Autodesk Inventor part; units mm, degrees
(part 2 of 3)
  line L844 (-43.6734, 26.1204) -> (-43.9834, 26.1204) projected
  line L845 (-43.9834, 26.1204) -> (-43.9834, 25.7204) projected
  line L846 (-43.9834, 25.7204) -> (-43.6734, 25.7204) projected
  line L847 (-43.6734, 25.7204) -> (-43.6734, 25.3204) projected
  line L848 (-43.6734, 25.3204) -> (-43.9834, 25.3204) projected
  line L849 (-43.9834, 25.3204) -> (-43.9834, 24.9204) projected
  line L850 (-43.9834, 24.9204) -> (-43.6734, 24.9204) projected
  line L851 (-43.6734, 24.9204) -> (-43.6734, 24.5204) projected
  line L852 (-43.6734, 24.5204) -> (-43.9834, 24.5204) projected
  line L853 (-43.9834, 24.5204) -> (-43.9834, 24.1204) projected
  line L854 (-43.9834, 24.1204) -> (-43.6734, 24.1204) projected
  line L855 (-43.6734, 24.1204) -> (-43.6734, 23.7204) projected
  line L856 (-43.6734, 23.7204) -> (-43.9834, 23.7204) projected
  line L857 (-43.9834, 23.7204) -> (-43.9834, 23.4704) projected
  arc A41 (-44.5384, 22.5149) -> (-43.9834, 23.4704) centre (-45.0834, 23.4704) ccw projected
  line L858 (-44.5384, 22.5149) -> (-44.5384, 22.4454) projected
  line L859 (-44.5384, 22.4454) -> (-44.6842, 22.4454) projected
  line L860 (-25.2834, -31.9046) -> (-25.2834, -32.3046) projected
  line L861 (-25.2834, -32.3046) -> (-24.6634, -32.3046) projected
  line L862 (-24.6634, -32.3046) -> (-24.6634, -32.7046) projected
  line L863 (-24.6634, -32.7046) -> (-25.286, -32.7046) projected
  arc A42 (-25.5349, -33.3296) -> (-25.286, -32.7046) centre (-26.3834, -32.6296) ccw projected
  line L864 (-25.5349, -33.3296) -> (-25.5284, -33.3296) projected
  line L865 (-25.5284, -33.3296) -> (-25.5284, -33.9796) projected
  line L866 (-25.5284, -33.9796) -> (-27.1284, -33.9796) projected
  line L867 (-27.1284, -33.9796) -> (-27.1284, -33.4389) projected
  arc A43 (-27.4808, -32.7046) -> (-27.1284, -33.4389) centre (-26.3834, -32.6296) ccw projected
  line L868 (-27.4808, -32.7046) -> (-27.9934, -32.7046) projected
  line L869 (-27.9934, -32.7046) -> (-27.9934, -32.3046) projected
  line L870 (-27.9934, -32.3046) -> (-27.4834, -32.3046) projected
  line L871 (-27.4834, -32.3046) -> (-27.4834, -31.9046) projected
  line L872 (-27.4834, -31.9046) -> (-27.9934, -31.9046) projected
  line L873 (-27.9934, -31.9046) -> (-27.9934, -31.5046) projected
  line L874 (-27.9934, -31.5046) -> (-27.4834, -31.5046) projected
  line L875 (-27.4834, -31.5046) -> (-27.4834, -31.1046) projected
  line L876 (-27.4834, -31.1046) -> (-27.9934, -31.1046) projected
  line L877 (-27.9934, -31.1046) -> (-27.9934, -30.7046) projected
  line L878 (-27.9934, -30.7046) -> (-27.4834, -30.7046) projected
  line L879 (-27.4834, -30.7046) -> (-27.4834, -30.3046) projected
  line L880 (-27.4834, -30.3046) -> (-27.9934, -30.3046) projected
  line L881 (-27.9934, -30.3046) -> (-27.9934, -29.9046) projected
  line L882 (-27.9934, -29.9046) -> (-27.4834, -29.9046) projected
  line L883 (-27.4834, -29.9046) -> (-27.4834, -29.5046) projected
  line L884 (-27.4834, -29.5046) -> (-27.9934, -29.5046) projected
  line L885 (-27.9934, -29.5046) -> (-27.9934, -29.1046) projected
  line L886 (-27.9934, -29.1046) -> (-27.4834, -29.1046) projected
  line L887 (-27.4834, -29.1046) -> (-27.4834, -28.7046) projected
  line L888 (-27.4834, -28.7046) -> (-27.9934, -28.7046) projected
  line L889 (-27.9934, -28.7046) -> (-27.9934, -28.3046) projected
  line L890 (-27.9934, -28.3046) -> (-27.4834, -28.3046) projected
  line L891 (-27.4834, -28.3046) -> (-27.4834, -27.9046) projected
  line L892 (-27.4834, -27.9046) -> (-27.9934, -27.9046) projected
  line L893 (-27.9934, -27.9046) -> (-27.9934, -27.5046) projected
  line L894 (-27.9934, -27.5046) -> (-27.4834, -27.5046) projected
  line L895 (-27.4834, -27.5046) -> (-27.4834, -27.1046) projected
  line L896 (-27.4834, -27.1046) -> (-27.9934, -27.1046) projected
  line L897 (-27.9934, -27.1046) -> (-27.9934, -26.7046) projected
  line L898 (-27.9934, -26.7046) -> (-27.4831, -26.7046) projected
  arc A44 (-27.1284, -25.9203) -> (-27.4831, -26.7046) centre (-26.3834, -26.7296) ccw projected
  line L899 (-27.1284, -25.9203) -> (-27.1284, -25.4296) projected
  line L900 (-27.1284, -25.4296) -> (-25.5284, -25.4296) projected
  line L901 (-25.5284, -25.4296) -> (-25.5284, -26.0375) projected
  arc A45 (-25.2837, -26.7046) -> (-25.5284, -26.0375) centre (-26.3834, -26.7296) ccw projected
  line L902 (-25.2837, -26.7046) -> (-24.6634, -26.7046) projected
  line L903 (-24.6634, -26.7046) -> (-24.6634, -27.1046) projected
  line L904 (-24.6634, -27.1046) -> (-25.2834, -27.1046) projected
  line L905 (-25.2834, -27.1046) -> (-25.2834, -27.5046) projected
  line L906 (-25.2834, -27.5046) -> (-24.6634, -27.5046) projected
  line L907 (-24.6634, -27.5046) -> (-24.6634, -27.9046) projected
  line L908 (-24.6634, -27.9046) -> (-25.2834, -27.9046) projected
  line L909 (-25.2834, -27.9046) -> (-25.2834, -28.3046) projected
  line L910 (-25.2834, -28.3046) -> (-24.6634, -28.3046) projected
  line L911 (-24.6634, -28.3046) -> (-24.6634, -28.7046) projected
  line L912 (-24.6634, -28.7046) -> (-25.2834, -28.7046) projected
  line L913 (-25.2834, -28.7046) -> (-25.2834, -29.1046) projected
  line L914 (-25.2834, -29.1046) -> (-24.6634, -29.1046) projected
  line L915 (-24.6634, -29.1046) -> (-24.6634, -29.5046) projected
  line L916 (-24.6634, -29.5046) -> (-25.2834, -29.5046) projected
  line L917 (-25.2834, -29.5046) -> (-25.2834, -29.9046) projected
  line L918 (-25.2834, -29.9046) -> (-24.6634, -29.9046) projected
  line L919 (-24.6634, -29.9046) -> (-24.6634, -30.3046) projected
  line L920 (-24.6634, -30.3046) -> (-25.2834, -30.3046) projected
  line L921 (-25.2834, -30.3046) -> (-25.2834, -30.7046) projected
  line L922 (-25.2834, -30.7046) -> (-24.6634, -30.7046) projected
  line L923 (-24.6634, -30.7046) -> (-24.6634, -31.1046) projected
  line L924 (-24.6634, -31.1046) -> (-25.2834, -31.1046) projected
  line L925 (-25.2834, -31.1046) -> (-25.2834, -31.5046) projected
  line L926 (-25.2834, -31.5046) -> (-24.6634, -31.5046) projected
  line L927 (-24.6634, -31.5046) -> (-24.6634, -31.9046) projected
  line L928 (-24.6634, -31.9046) -> (-25.2834, -31.9046) projected
  arc A46 (-26.6166, 3.6954) -> (-26.1502, 3.6954) centre (-26.3834, 4.7704) ccw projected
  line L929 (-26.6166, 3.6954) -> (-27.2859, 3.6954) projected
  line L930 (-27.2859, 3.6954) -> (-27.2859, 4.1415) projected
  arc A47 (-27.4834, 4.7704) -> (-27.2859, 4.1415) centre (-26.3834, 4.7704) ccw projected
  line L931 (-27.4834, 4.7704) -> (-27.4834, 4.9704) projected
  line L932 (-27.4834, 4.9704) -> (-28.1509, 4.9704) projected
  line L933 (-28.1509, 4.9704) -> (-28.1509, 5.3704) projected
  line L934 (-28.1509, 5.3704) -> (-27.4834, 5.3704) projected
  line L935 (-27.4834, 5.3704) -> (-27.4834, 5.7704) projected
  line L936 (-27.4834, 5.7704) -> (-28.1509, 5.7704) projected
  line L937 (-28.1509, 5.7704) -> (-28.1509, 6.1704) projected
  line L938 (-28.1509, 6.1704) -> (-27.4834, 6.1704) projected
  line L939 (-27.4834, 6.1704) -> (-27.4834, 6.5704) projected
  line L940 (-27.4834, 6.5704) -> (-28.1509, 6.5704) projected
  line L941 (-28.1509, 6.5704) -> (-28.1509, 6.9704) projected
  line L942 (-28.1509, 6.9704) -> (-27.4834, 6.9704) projected
  line L943 (-27.4834, 6.9704) -> (-27.4834, 7.3704) projected
  line L944 (-27.4834, 7.3704) -> (-28.1509, 7.3704) projected
  line L945 (-28.1509, 7.3704) -> (-28.1509, 7.7704) projected
  line L946 (-28.1509, 7.7704) -> (-27.4834, 7.7704) projected
  line L947 (-27.4834, 7.7704) -> (-27.4834, 8.1704) projected
  line L948 (-27.4834, 8.1704) -> (-28.1509, 8.1704) projected
  line L949 (-28.1509, 8.1704) -> (-28.1509, 8.5704) projected
  line L950 (-28.1509, 8.5704) -> (-27.4834, 8.5704) projected
  line L951 (-27.4834, 8.5704) -> (-27.4834, 8.9704) projected
  line L952 (-27.4834, 8.9704) -> (-28.1509, 8.9704) projected
  line L953 (-28.1509, 8.9704) -> (-28.1509, 9.3704) projected
  line L954 (-28.1509, 9.3704) -> (-27.4834, 9.3704) projected
  line L955 (-27.4834, 9.3704) -> (-27.4834, 9.7704) projected
  line L956 (-27.4834, 9.7704) -> (-28.1509, 9.7704) projected
  line L957 (-28.1509, 9.7704) -> (-28.1509, 10.1704) projected
  line L958 (-28.1509, 10.1704) -> (-27.4834, 10.1704) projected
  line L959 (-27.4834, 10.1704) -> (-27.4834, 10.5704) projected
  line L960 (-27.4834, 10.5704) -> (-28.1509, 10.5704) projected
  line L961 (-28.1509, 10.5704) -> (-28.1509, 10.9704) projected
  line L962 (-28.1509, 10.9704) -> (-27.4417, 10.9704) projected
  arc A48 (-26.9787, 11.5954) -> (-27.4417, 10.9704) centre (-26.3834, 10.6704) ccw projected
  line L963 (-26.9787, 11.5954) -> (-27.2859, 11.5954) projected
  line L964 (-27.2859, 11.5954) -> (-27.2859, 12.2454) projected
  line L965 (-27.2859, 12.2454) -> (-25.6859, 12.2454) projected
  line L966 (-25.6859, 12.2454) -> (-25.6859, 11.5954) projected
  line L967 (-25.6859, 11.5954) -> (-25.7881, 11.5954) projected
  arc A49 (-25.3251, 10.9704) -> (-25.7881, 11.5954) centre (-26.3834, 10.6704) ccw projected
  line L968 (-25.3251, 10.9704) -> (-24.8209, 10.9704) projected
  line L969 (-24.8209, 10.9704) -> (-24.8209, 10.5704) projected
  line L970 (-24.8209, 10.5704) -> (-25.2834, 10.5704) projected
  line L971 (-25.2834, 10.5704) -> (-25.2834, 10.1704) projected
  line L972 (-25.2834, 10.1704) -> (-24.8209, 10.1704) projected
  line L973 (-24.8209, 10.1704) -> (-24.8209, 9.7704) projected
  line L974 (-24.8209, 9.7704) -> (-25.2834, 9.7704) projected
  line L975 (-25.2834, 9.7704) -> (-25.2834, 9.3704) projected
  line L976 (-25.2834, 9.3704) -> (-24.8209, 9.3704) projected
  line L977 (-24.8209, 9.3704) -> (-24.8209, 8.9704) projected
  line L978 (-24.8209, 8.9704) -> (-25.2834, 8.9704) projected
  line L979 (-25.2834, 8.9704) -> (-25.2834, 8.5704) projected
  line L980 (-25.2834, 8.5704) -> (-24.8209, 8.5704) projected
  line L981 (-24.8209, 8.5704) -> (-24.8209, 8.1704) projected
  line L982 (-24.8209, 8.1704) -> (-25.2834, 8.1704) projected
  line L983 (-25.2834, 8.1704) -> (-25.2834, 7.7704) projected
  line L984 (-25.2834, 7.7704) -> (-24.8209, 7.7704) projected
  line L985 (-24.8209, 7.7704) -> (-24.8209, 7.3704) projected
  line L986 (-24.8209, 7.3704) -> (-25.2834, 7.3704) projected
  line L987 (-25.2834, 7.3704) -> (-25.2834, 6.9704) projected
  line L988 (-25.2834, 6.9704) -> (-24.8209, 6.9704) projected
  line L989 (-24.8209, 6.9704) -> (-24.8209, 6.5704) projected
  line L990 (-24.8209, 6.5704) -> (-25.2834, 6.5704) projected
  line L991 (-25.2834, 6.5704) -> (-25.2834, 6.1704) projected
  line L992 (-25.2834, 6.1704) -> (-24.8209, 6.1704) projected
  line L993 (-24.8209, 6.1704) -> (-24.8209, 5.7704) projected
  line L994 (-24.8209, 5.7704) -> (-25.2834, 5.7704) projected
  line L995 (-25.2834, 5.7704) -> (-25.2834, 5.3704) projected
  line L996 (-25.2834, 5.3704) -> (-24.8209, 5.3704) projected
  line L997 (-24.8209, 5.3704) -> (-24.8209, 4.9704) projected
  line L998 (-24.8209, 4.9704) -> (-25.2834, 4.9704) projected
  line L999 (-25.2834, 4.9704) -> (-25.2834, 4.7704) projected
  arc A50 (-25.6859, 3.9198) -> (-25.2834, 4.7704) centre (-26.3834, 4.7704) ccw projected
  line L1000 (-25.6859, 3.9198) -> (-25.6859, 3.6954) projected
  line L1001 (-25.6859, 3.6954) -> (-26.1502, 3.6954) projected
  arc A51 (-26.7113, 22.4204) -> (-26.0555, 22.4204) centre (-26.3834, 23.4704) ccw projected
  line L1002 (-26.7113, 22.4204) -> (-27.0884, 22.4204) projected
  line L1003 (-27.0884, 22.4204) -> (-27.0884, 22.626) projected
  arc A52 (-27.4834, 23.4704) -> (-27.0884, 22.626) centre (-26.3834, 23.4704) ccw projected
  line L1004 (-27.4834, 23.4704) -> (-27.4834, 23.6954) projected
  line L1005 (-27.4834, 23.6954) -> (-27.9534, 23.6954) projected
  line L1006 (-27.9534, 23.6954) -> (-27.9534, 24.0954) projected
  line L1007 (-27.9534, 24.0954) -> (-27.4834, 24.0954) projected
  line L1008 (-27.4834, 24.0954) -> (-27.4834, 24.4954) projected
  line L1009 (-27.4834, 24.4954) -> (-27.9534, 24.4954) projected
  line L1010 (-27.9534, 24.4954) -> (-27.9534, 24.8954) projected
  line L1011 (-27.9534, 24.8954) -> (-27.4834, 24.8954) projected
  line L1012 (-27.4834, 24.8954) -> (-27.4834, 25.2954) projected
  line L1013 (-27.4834, 25.2954) -> (-27.9534, 25.2954) projected
  line L1014 (-27.9534, 25.2954) -> (-27.9534, 25.6954) projected
  line L1015 (-27.9534, 25.6954) -> (-27.4834, 25.6954) projected
  line L1016 (-27.4834, 25.6954) -> (-27.4834, 26.0954) projected
  line L1017 (-27.4834, 26.0954) -> (-27.9534, 26.0954) projected
  line L1018 (-27.9534, 26.0954) -> (-27.9534, 26.4954) projected
  line L1019 (-27.9534, 26.4954) -> (-27.4834, 26.4954) projected
  line L1020 (-27.4834, 26.4954) -> (-27.4834, 26.8954) projected
  line L1021 (-27.4834, 26.8954) -> (-27.9534, 26.8954) projected
  line L1022 (-27.9534, 26.8954) -> (-27.9534, 27.2954) projected
  line L1023 (-27.9534, 27.2954) -> (-27.4834, 27.2954) projected
  line L1024 (-27.4834, 27.2954) -> (-27.4834, 27.6954) projected
  line L1025 (-27.4834, 27.6954) -> (-27.9534, 27.6954) projected
  line L1026 (-27.9534, 27.6954) -> (-27.9534, 28.0954) projected
  line L1027 (-27.9534, 28.0954) -> (-27.4834, 28.0954) projected
  line L1028 (-27.4834, 28.0954) -> (-27.4834, 28.4954) projected
  line L1029 (-27.4834, 28.4954) -> (-27.9534, 28.4954) projected
  line L1030 (-27.9534, 28.4954) -> (-27.9534, 28.8954) projected
  line L1031 (-27.9534, 28.8954) -> (-27.4834, 28.8954) projected
  line L1032 (-27.4834, 28.8954) -> (-27.4834, 29.2954) projected
  line L1033 (-27.4834, 29.2954) -> (-27.9534, 29.2954) projected
  line L1034 (-27.9534, 29.2954) -> (-27.9534, 29.6954) projected
  line L1035 (-27.9534, 29.6954) -> (-27.4343, 29.6954) projected
  arc A53 (-26.9379, 30.3204) -> (-27.4343, 29.6954) centre (-26.3834, 29.3704) ccw projected
  line L1036 (-26.9379, 30.3204) -> (-27.0884, 30.3204) projected
  line L1037 (-27.0884, 30.3204) -> (-27.0884, 30.9704) projected
  line L1038 (-27.0884, 30.9704) -> (-25.4884, 30.9704) projected
  line L1039 (-25.4884, 30.9704) -> (-25.4884, 30.3204) projected
  line L1040 (-25.4884, 30.3204) -> (-25.8289, 30.3204) projected
  arc A54 (-25.3325, 29.6954) -> (-25.8289, 30.3204) centre (-26.3834, 29.3704) ccw projected
  line L1041 (-25.3325, 29.6954) -> (-24.6234, 29.6954) projected
  line L1042 (-24.6234, 29.6954) -> (-24.6234, 29.2954) projected
  line L1043 (-24.6234, 29.2954) -> (-25.2834, 29.2954) projected
  line L1044 (-25.2834, 29.2954) -> (-25.2834, 28.8954) projected
  line L1045 (-25.2834, 28.8954) -> (-24.6234, 28.8954) projected
  line L1046 (-24.6234, 28.8954) -> (-24.6234, 28.4954) projected
  line L1047 (-24.6234, 28.4954) -> (-25.2834, 28.4954) projected
  line L1048 (-25.2834, 28.4954) -> (-25.2834, 28.0954) projected
  line L1049 (-25.2834, 28.0954) -> (-24.6234, 28.0954) projected
  line L1050 (-24.6234, 28.0954) -> (-24.6234, 27.6954) projected
  line L1051 (-24.6234, 27.6954) -> (-25.2834, 27.6954) projected
  line L1052 (-25.2834, 27.6954) -> (-25.2834, 27.2954) projected
  line L1053 (-25.2834, 27.2954) -> (-24.6234, 27.2954) projected
  line L1054 (-24.6234, 27.2954) -> (-24.6234, 26.8954) projected
  line L1055 (-24.6234, 26.8954) -> (-25.2834, 26.8954) projected
  line L1056 (-25.2834, 26.8954) -> (-25.2834, 26.4954) projected
  line L1057 (-25.2834, 26.4954) -> (-24.6234, 26.4954) projected
  line L1058 (-24.6234, 26.4954) -> (-24.6234, 26.0954) projected
  line L1059 (-24.6234, 26.0954) -> (-25.2834, 26.0954) projected
  line L1060 (-25.2834, 26.0954) -> (-25.2834, 25.6954) projected
  line L1061 (-25.2834, 25.6954) -> (-24.6234, 25.6954) projected
  line L1062 (-24.6234, 25.6954) -> (-24.6234, 25.2954) projected
  line L1063 (-24.6234, 25.2954) -> (-25.2834, 25.2954) projected
  line L1064 (-25.2834, 25.2954) -> (-25.2834, 24.8954) projected
  line L1065 (-25.2834, 24.8954) -> (-24.6234, 24.8954) projected
  line L1066 (-24.6234, 24.8954) -> (-24.6234, 24.4954) projected
  line L1067 (-24.6234, 24.4954) -> (-25.2834, 24.4954) projected
  line L1068 (-25.2834, 24.4954) -> (-25.2834, 24.0954) projected
  line L1069 (-25.2834, 24.0954) -> (-24.6234, 24.0954) projected
  line L1070 (-24.6234, 24.0954) -> (-24.6234, 23.6954) projected
  line L1071 (-24.6234, 23.6954) -> (-25.2834, 23.6954) projected
  line L1072 (-25.2834, 23.6954) -> (-25.2834, 23.4704) projected
  arc A55 (-25.4884, 22.8309) -> (-25.2834, 23.4704) centre (-26.3834, 23.4704) ccw projected
  line L1073 (-25.4884, 22.8309) -> (-25.4884, 22.4204) projected
  line L1074 (-25.4884, 22.4204) -> (-26.0555, 22.4204) projected
  line L1075 (-6.5834, -31.8296) -> (-6.5834, -32.2296) projected
  line L1076 (-6.5834, -32.2296) -> (-5.8559, -32.2296) projected
  line L1077 (-5.8559, -32.2296) -> (-5.8559, -32.6296) projected
  line L1078 (-5.8559, -32.6296) -> (-6.5834, -32.6296) projected
  arc A56 (-6.7782, -33.2546) -> (-6.5834, -32.6296) centre (-7.6834, -32.6296) ccw projected
  line L1079 (-6.7782, -33.2546) -> (-6.7209, -33.2546) projected
  line L1080 (-6.7209, -33.2546) -> (-6.7209, -33.9046) projected
  line L1081 (-6.7209, -33.9046) -> (-8.3209, -33.9046) projected
  line L1082 (-8.3209, -33.9046) -> (-8.3209, -33.526) projected
  arc A57 (-8.7834, -32.6296) -> (-8.3209, -33.526) centre (-7.6834, -32.6296) ccw projected
  line L1083 (-8.7834, -32.6296) -> (-9.1859, -32.6296) projected
  line L1084 (-9.1859, -32.6296) -> (-9.1859, -32.2296) projected
  line L1085 (-9.1859, -32.2296) -> (-8.7834, -32.2296) projected
  line L1086 (-8.7834, -32.2296) -> (-8.7834, -31.8296) projected
  line L1087 (-8.7834, -31.8296) -> (-9.1859, -31.8296) projected
  line L1088 (-9.1859, -31.8296) -> (-9.1859, -31.4296) projected
  line L1089 (-9.1859, -31.4296) -> (-8.7834, -31.4296) projected
  line L1090 (-8.7834, -31.4296) -> (-8.7834, -31.0296) projected
  line L1091 (-8.7834, -31.0296) -> (-9.1859, -31.0296) projected
  line L1092 (-9.1859, -31.0296) -> (-9.1859, -30.6296) projected
  line L1093 (-9.1859, -30.6296) -> (-8.7834, -30.6296) projected
  line L1094 (-8.7834, -30.6296) -> (-8.7834, -30.2296) projected
  line L1095 (-8.7834, -30.2296) -> (-9.1859, -30.2296) projected
  line L1096 (-9.1859, -30.2296) -> (-9.1859, -29.8296) projected
  line L1097 (-9.1859, -29.8296) -> (-8.7834, -29.8296) projected
  line L1098 (-8.7834, -29.8296) -> (-8.7834, -29.4296) projected
  line L1099 (-8.7834, -29.4296) -> (-9.1859, -29.4296) projected
  line L1100 (-9.1859, -29.4296) -> (-9.1859, -29.0296) projected
  line L1101 (-9.1859, -29.0296) -> (-8.7834, -29.0296) projected
  line L1102 (-8.7834, -29.0296) -> (-8.7834, -28.6296) projected
  line L1103 (-8.7834, -28.6296) -> (-9.1859, -28.6296) projected
  line L1104 (-9.1859, -28.6296) -> (-9.1859, -28.2296) projected
  line L1105 (-9.1859, -28.2296) -> (-8.7834, -28.2296) projected
  line L1106 (-8.7834, -28.2296) -> (-8.7834, -27.8296) projected
  line L1107 (-8.7834, -27.8296) -> (-9.1859, -27.8296) projected
  line L1108 (-9.1859, -27.8296) -> (-9.1859, -27.4296) projected
  line L1109 (-9.1859, -27.4296) -> (-8.7834, -27.4296) projected
  line L1110 (-8.7834, -27.4296) -> (-8.7834, -27.0296) projected
  line L1111 (-8.7834, -27.0296) -> (-9.1859, -27.0296) projected
  line L1112 (-9.1859, -27.0296) -> (-9.1859, -26.6296) projected
  line L1113 (-9.1859, -26.6296) -> (-8.7788, -26.6296) projected
  arc A58 (-8.3209, -25.8332) -> (-8.7788, -26.6296) centre (-7.6834, -26.7296) ccw projected
  line L1114 (-8.3209, -25.8332) -> (-8.3209, -25.3546) projected
  line L1115 (-8.3209, -25.3546) -> (-6.7209, -25.3546) projected
  line L1116 (-6.7209, -25.3546) -> (-6.7209, -26.0046) projected
  line L1117 (-6.7209, -26.0046) -> (-6.8561, -26.0046) projected
  arc A59 (-6.588, -26.6296) -> (-6.8561, -26.0046) centre (-7.6834, -26.7296) ccw projected
  line L1118 (-6.588, -26.6296) -> (-5.8559, -26.6296) projected
  line L1119 (-5.8559, -26.6296) -> (-5.8559, -27.0296) projected
  line L1120 (-5.8559, -27.0296) -> (-6.5834, -27.0296) projected
  line L1121 (-6.5834, -27.0296) -> (-6.5834, -27.4296) projected
  line L1122 (-6.5834, -27.4296) -> (-5.8559, -27.4296) projected
  line L1123 (-5.8559, -27.4296) -> (-5.8559, -27.8296) projected
  line L1124 (-5.8559, -27.8296) -> (-6.5834, -27.8296) projected
  line L1125 (-6.5834, -27.8296) -> (-6.5834, -28.2296) projected
  line L1126 (-6.5834, -28.2296) -> (-5.8559, -28.2296) projected
  line L1127 (-5.8559, -28.2296) -> (-5.8559, -28.6296) projected
  line L1128 (-5.8559, -28.6296) -> (-6.5834, -28.6296) projected
  line L1129 (-6.5834, -28.6296) -> (-6.5834, -29.0296) projected
  line L1130 (-6.5834, -29.0296) -> (-5.8559, -29.0296) projected
  line L1131 (-5.8559, -29.0296) -> (-5.8559, -29.4296) projected
  line L1132 (-5.8559, -29.4296) -> (-6.5834, -29.4296) projected
  line L1133 (-6.5834, -29.4296) -> (-6.5834, -29.8296) projected
  line L1134 (-6.5834, -29.8296) -> (-5.8559, -29.8296) projected
  line L1135 (-5.8559, -29.8296) -> (-5.8559, -30.2296) projected
  line L1136 (-5.8559, -30.2296) -> (-6.5834, -30.2296) projected
  line L1137 (-6.5834, -30.2296) -> (-6.5834, -30.6296) projected
  line L1138 (-6.5834, -30.6296) -> (-5.8559, -30.6296) projected
  line L1139 (-5.8559, -30.6296) -> (-5.8559, -31.0296) projected
  line L1140 (-5.8559, -31.0296) -> (-6.5834, -31.0296) projected
  line L1141 (-6.5834, -31.0296) -> (-6.5834, -31.4296) projected
  line L1142 (-6.5834, -31.4296) -> (-5.8559, -31.4296) projected
  line L1143 (-5.8559, -31.4296) -> (-5.8559, -31.8296) projected
  line L1144 (-5.8559, -31.8296) -> (-6.5834, -31.8296) projected
  arc A60 (-8.1417, 3.7704) -> (-7.2251, 3.7704) centre (-7.6834, 4.7704) ccw projected
  line L1145 (-8.1417, 3.7704) -> (-8.4784, 3.7704) projected
  line L1146 (-8.4784, 3.7704) -> (-8.4784, 4.0102) projected
  arc A61 (-8.7834, 4.7704) -> (-8.4784, 4.0102) centre (-7.6834, 4.7704) ccw projected
  line L1147 (-8.7834, 4.7704) -> (-8.7834, 5.0454) projected
  line L1148 (-8.7834, 5.0454) -> (-9.3434, 5.0454) projected
  line L1149 (-9.3434, 5.0454) -> (-9.3434, 5.4454) projected
  line L1150 (-9.3434, 5.4454) -> (-8.7834, 5.4454) projected
  line L1151 (-8.7834, 5.4454) -> (-8.7834, 5.8454) projected
  line L1152 (-8.7834, 5.8454) -> (-9.3434, 5.8454) projected
  line L1153 (-9.3434, 5.8454) -> (-9.3434, 6.2454) projected
  line L1154 (-9.3434, 6.2454) -> (-8.7834, 6.2454) projected
  line L1155 (-8.7834, 6.2454) -> (-8.7834, 6.6454) projected
  line L1156 (-8.7834, 6.6454) -> (-9.3434, 6.6454) projected
  line L1157 (-9.3434, 6.6454) -> (-9.3434, 7.0454) projected
  line L1158 (-9.3434, 7.0454) -> (-8.7834, 7.0454) projected
  line L1159 (-8.7834, 7.0454) -> (-8.7834, 7.4454) projected
  line L1160 (-8.7834, 7.4454) -> (-9.3434, 7.4454) projected
  line L1161 (-9.3434, 7.4454) -> (-9.3434, 7.8454) projected
  line L1162 (-9.3434, 7.8454) -> (-8.7834, 7.8454) projected
  line L1163 (-8.7834, 7.8454) -> (-8.7834, 8.2454) projected
  line L1164 (-8.7834, 8.2454) -> (-9.3434, 8.2454) projected
  line L1165 (-9.3434, 8.2454) -> (-9.3434, 8.6454) projected
  line L1166 (-9.3434, 8.6454) -> (-8.7834, 8.6454) projected
  line L1167 (-8.7834, 8.6454) -> (-8.7834, 9.0454) projected
  line L1168 (-8.7834, 9.0454) -> (-9.3434, 9.0454) projected
  line L1169 (-9.3434, 9.0454) -> (-9.3434, 9.4454) projected
  line L1170 (-9.3434, 9.4454) -> (-8.7834, 9.4454) projected
  line L1171 (-8.7834, 9.4454) -> (-8.7834, 9.8454) projected
  line L1172 (-8.7834, 9.8454) -> (-9.3434, 9.8454) projected
  line L1173 (-9.3434, 9.8454) -> (-9.3434, 10.2454) projected
  line L1174 (-9.3434, 10.2454) -> (-8.7834, 10.2454) projected
  line L1175 (-8.7834, 10.2454) -> (-8.7834, 10.6454) projected
  line L1176 (-8.7834, 10.6454) -> (-9.3434, 10.6454) projected
  line L1177 (-9.3434, 10.6454) -> (-9.3434, 11.0454) projected
  line L1178 (-9.3434, 11.0454) -> (-8.7175, 11.0454) projected
  arc A62 (-8.1417, 11.6704) -> (-8.7175, 11.0454) centre (-7.6834, 10.6704) ccw projected
  line L1179 (-8.1417, 11.6704) -> (-8.4784, 11.6704) projected
  line L1180 (-8.4784, 11.6704) -> (-8.4784, 12.3204) projected
  line L1181 (-8.4784, 12.3204) -> (-6.8784, 12.3204) projected
  line L1182 (-6.8784, 12.3204) -> (-6.8784, 11.6704) projected
  line L1183 (-6.8784, 11.6704) -> (-7.2251, 11.6704) projected
  arc A63 (-6.6493, 11.0454) -> (-7.2251, 11.6704) centre (-7.6834, 10.6704) ccw projected
  line L1184 (-6.6493, 11.0454) -> (-6.0134, 11.0454) projected
  line L1185 (-6.0134, 11.0454) -> (-6.0134, 10.6454) projected
  line L1186 (-6.0134, 10.6454) -> (-6.5834, 10.6454) projected
  line L1187 (-6.5834, 10.6454) -> (-6.5834, 10.2454) projected
  line L1188 (-6.5834, 10.2454) -> (-6.0134, 10.2454) projected
  line L1189 (-6.0134, 10.2454) -> (-6.0134, 9.8454) projected
  line L1190 (-6.0134, 9.8454) -> (-6.5834, 9.8454) projected
  line L1191 (-6.5834, 9.8454) -> (-6.5834, 9.4454) projected
  line L1192 (-6.5834, 9.4454) -> (-6.0134, 9.4454) projected
  line L1193 (-6.0134, 9.4454) -> (-6.0134, 9.0454) projected
  line L1194 (-6.0134, 9.0454) -> (-6.5834, 9.0454) projected
  line L1195 (-6.5834, 9.0454) -> (-6.5834, 8.6454) projected
  line L1196 (-6.5834, 8.6454) -> (-6.0134, 8.6454) projected
  line L1197 (-6.0134, 8.6454) -> (-6.0134, 8.2454) projected
  line L1198 (-6.0134, 8.2454) -> (-6.5834, 8.2454) projected
  line L1199 (-6.5834, 8.2454) -> (-6.5834, 7.8454) projected
  line L1200 (-6.5834, 7.8454) -> (-6.0134, 7.8454) projected
  line L1201 (-6.0134, 7.8454) -> (-6.0134, 7.4454) projected
  line L1202 (-6.0134, 7.4454) -> (-6.5834, 7.4454) projected
  line L1203 (-6.5834, 7.4454) -> (-6.5834, 7.0454) projected
  line L1204 (-6.5834, 7.0454) -> (-6.0134, 7.0454) projected
  line L1205 (-6.0134, 7.0454) -> (-6.0134, 6.6454) projected
  line L1206 (-6.0134, 6.6454) -> (-6.5834, 6.6454) projected
  line L1207 (-6.5834, 6.6454) -> (-6.5834, 6.2454) projected
  line L1208 (-6.5834, 6.2454) -> (-6.0134, 6.2454) projected
  line L1209 (-6.0134, 6.2454) -> (-6.0134, 5.8454) projected
  line L1210 (-6.0134, 5.8454) -> (-6.5834, 5.8454) projected
  line L1211 (-6.5834, 5.8454) -> (-6.5834, 5.4454) projected
  line L1212 (-6.5834, 5.4454) -> (-6.0134, 5.4454) projected
  line L1213 (-6.0134, 5.4454) -> (-6.0134, 5.0454) projected
  line L1214 (-6.0134, 5.0454) -> (-6.5834, 5.0454) projected
  line L1215 (-6.5834, 5.0454) -> (-6.5834, 4.7704) projected
  arc A64 (-6.8784, 4.0208) -> (-6.5834, 4.7704) centre (-7.6834, 4.7704) ccw projected
  line L1216 (-6.8784, 4.0208) -> (-6.8784, 3.7704) projected
  line L1217 (-6.8784, 3.7704) -> (-7.2251, 3.7704) projected
  line L1218 (-8.7834, 28.7954) -> (-8.7834, 29.1954) projected
  line L1219 (-8.7834, 29.1954) -> (-9.1284, 29.1954) projected
  line L1220 (-9.1284, 29.1954) -> (-9.1284, 29.5954) projected
  line L1221 (-9.1284, 29.5954) -> (-8.7601, 29.5954) projected
  arc A65 (-8.2634, 30.3051) -> (-8.7601, 29.5954) centre (-7.6834, 29.3704) ccw projected
  line L1222 (-8.2634, 30.3051) -> (-8.2634, 30.8704) projected
  line L1223 (-8.2634, 30.8704) -> (-6.6634, 30.8704) projected
  line L1224 (-6.6634, 30.8704) -> (-6.6634, 30.2204) projected
  line L1225 (-6.6634, 30.2204) -> (-6.9852, 30.2204) projected
  arc A66 (-6.5884, 29.4752) -> (-6.9852, 30.2204) centre (-7.6834, 29.3704) ccw projected
  line L1226 (-6.5884, 29.4752) -> (-6.5884, 29.5954) projected
  line L1227 (-6.5884, 29.5954) -> (-5.7984, 29.5954) projected
  line L1228 (-5.7984, 29.5954) -> (-5.7984, 29.1954) projected
  line L1229 (-5.7984, 29.1954) -> (-6.5834, 29.1954) projected
  line L1230 (-6.5834, 29.1954) -> (-6.5834, 28.7954) projected
  line L1231 (-6.5834, 28.7954) -> (-5.7984, 28.7954) projected
  line L1232 (-5.7984, 28.7954) -> (-5.7984, 28.3954) projected
  line L1233 (-5.7984, 28.3954) -> (-6.5834, 28.3954) projected
  line L1234 (-6.5834, 28.3954) -> (-6.5834, 27.9954) projected
  line L1235 (-6.5834, 27.9954) -> (-5.7984, 27.9954) projected
  line L1236 (-5.7984, 27.9954) -> (-5.7984, 27.5954) projected
  line L1237 (-5.7984, 27.5954) -> (-6.5834, 27.5954) projected
  line L1238 (-6.5834, 27.5954) -> (-6.5834, 27.1954) projected
  line L1239 (-6.5834, 27.1954) -> (-5.7984, 27.1954) projected
  line L1240 (-5.7984, 27.1954) -> (-5.7984, 26.7954) projected
  line L1241 (-5.7984, 26.7954) -> (-6.5834, 26.7954) projected
  line L1242 (-6.5834, 26.7954) -> (-6.5834, 26.3954) projected
  line L1243 (-6.5834, 26.3954) -> (-5.7984, 26.3954) projected
  line L1244 (-5.7984, 26.3954) -> (-5.7984, 25.9954) projected
  line L1245 (-5.7984, 25.9954) -> (-6.5834, 25.9954) projected
  line L1246 (-6.5834, 25.9954) -> (-6.5834, 25.5954) projected
  line L1247 (-6.5834, 25.5954) -> (-5.7984, 25.5954) projected
  line L1248 (-5.7984, 25.5954) -> (-5.7984, 25.1954) projected
  line L1249 (-5.7984, 25.1954) -> (-6.5834, 25.1954) projected
  line L1250 (-6.5834, 25.1954) -> (-6.5834, 24.7954) projected
  line L1251 (-6.5834, 24.7954) -> (-5.7984, 24.7954) projected
  line L1252 (-5.7984, 24.7954) -> (-5.7984, 24.3954) projected
  line L1253 (-5.7984, 24.3954) -> (-6.5834, 24.3954) projected
  line L1254 (-6.5834, 24.3954) -> (-6.5834, 23.9954) projected
  line L1255 (-6.5834, 23.9954) -> (-5.7984, 23.9954) projected
  line L1256 (-5.7984, 23.9954) -> (-5.7984, 23.5954) projected
  line L1257 (-5.7984, 23.5954) -> (-6.5834, 23.5954) projected
  line L1258 (-6.5834, 23.5954) -> (-6.5834, 23.4704) projected
  arc A67 (-6.7036, 22.9704) -> (-6.5834, 23.4704) centre (-7.6834, 23.4704) ccw projected
  line L1259 (-6.7036, 22.9704) -> (-6.6634, 22.9704) projected
  line L1260 (-6.6634, 22.9704) -> (-6.6634, 22.3204) projected
  line L1261 (-6.6634, 22.3204) -> (-8.2634, 22.3204) projected
  line L1262 (-8.2634, 22.3204) -> (-8.2634, 22.5357) projected
  arc A68 (-8.7834, 23.4704) -> (-8.2634, 22.5357) centre (-7.6834, 23.4704) ccw projected
  line L1263 (-8.7834, 23.4704) -> (-8.7834, 23.5954) projected
  line L1264 (-8.7834, 23.5954) -> (-9.1284, 23.5954) projected
  line L1265 (-9.1284, 23.5954) -> (-9.1284, 23.9954) projected
  line L1266 (-9.1284, 23.9954) -> (-8.7834, 23.9954) projected
  line L1267 (-8.7834, 23.9954) -> (-8.7834, 24.3954) projected
  line L1268 (-8.7834, 24.3954) -> (-9.1284, 24.3954) projected
  line L1269 (-9.1284, 24.3954) -> (-9.1284, 24.7954) projected
  line L1270 (-9.1284, 24.7954) -> (-8.7834, 24.7954) projected
  line L1271 (-8.7834, 24.7954) -> (-8.7834, 25.1954) projected
  line L1272 (-8.7834, 25.1954) -> (-9.1284, 25.1954) projected
  line L1273 (-9.1284, 25.1954) -> (-9.1284, 25.5954) projected
  line L1274 (-9.1284, 25.5954) -> (-8.7834, 25.5954) projected
  line L1275 (-8.7834, 25.5954) -> (-8.7834, 25.9954) projected
  line L1276 (-8.7834, 25.9954) -> (-9.1284, 25.9954) projected
  line L1277 (-9.1284, 25.9954) -> (-9.1284, 26.3954) projected
  line L1278 (-9.1284, 26.3954) -> (-8.7834, 26.3954) projected
  line L1279 (-8.7834, 26.3954) -> (-8.7834, 26.7954) projected
  line L1280 (-8.7834, 26.7954) -> (-9.1284, 26.7954) projected
  line L1281 (-9.1284, 26.7954) -> (-9.1284, 27.1954) projected
  line L1282 (-9.1284, 27.1954) -> (-8.7834, 27.1954) projected
  line L1283 (-8.7834, 27.1954) -> (-8.7834, 27.5954) projected
  line L1284 (-8.7834, 27.5954) -> (-9.1284, 27.5954) projected
  line L1285 (-9.1284, 27.5954) -> (-9.1284, 27.9954) projected
  line L1286 (-9.1284, 27.9954) -> (-8.7834, 27.9954) projected
  line L1287 (-8.7834, 27.9954) -> (-8.7834, 28.3954) projected
  line L1288 (-8.7834, 28.3954) -> (-9.1284, 28.3954) projected
  line L1289 (-9.1284, 28.3954) -> (-9.1284, 28.7954) projected
  line L1290 (-9.1284, 28.7954) -> (-8.7834, 28.7954) projected
  line L1291 (9.9166, -31.4296) -> (9.9166, -31.0296) projected
  line L1292 (9.9166, -31.0296) -> (9.6891, -31.0296) projected
  line L1293 (9.6891, -31.0296) -> (9.6891, -30.6296) projected
  line L1294 (9.6891, -30.6296) -> (9.9166, -30.6296) projected
  line L1295 (9.9166, -30.6296) -> (9.9166, -30.2296) projected
  line L1296 (9.9166, -30.2296) -> (9.6891, -30.2296) projected
  line L1297 (9.6891, -30.2296) -> (9.6891, -29.8296) projected
  line L1298 (9.6891, -29.8296) -> (9.9166, -29.8296) projected
  line L1299 (9.9166, -29.8296) -> (9.9166, -29.4296) projected
  line L1300 (9.9166, -29.4296) -> (9.6891, -29.4296) projected
  line L1301 (9.6891, -29.4296) -> (9.6891, -29.0296) projected
  line L1302 (9.6891, -29.0296) -> (9.9166, -29.0296) projected
  line L1303 (9.9166, -29.0296) -> (9.9166, -28.6296) projected
  line L1304 (9.9166, -28.6296) -> (9.6891, -28.6296) projected
  line L1305 (9.6891, -28.6296) -> (9.6891, -28.2296) projected
  line L1306 (9.6891, -28.2296) -> (9.9166, -28.2296) projected
  line L1307 (9.9166, -28.2296) -> (9.9166, -27.8296) projected
  line L1308 (9.9166, -27.8296) -> (9.6891, -27.8296) projected
  line L1309 (9.6891, -27.8296) -> (9.6891, -27.4296) projected
  line L1310 (9.6891, -27.4296) -> (9.9166, -27.4296) projected
  line L1311 (9.9166, -27.4296) -> (9.9166, -27.0296) projected
  line L1312 (9.9166, -27.0296) -> (9.6891, -27.0296) projected
  line L1313 (9.6891, -27.0296) -> (9.6891, -26.6296) projected
  line L1314 (9.6891, -26.6296) -> (9.9212, -26.6296) projected
  arc A69 (10.5541, -25.7316) -> (9.9212, -26.6296) centre (11.0166, -26.7296) ccw projected
  line L1315 (10.5541, -25.7316) -> (10.5541, -25.3546) projected
  line L1316 (10.5541, -25.3546) -> (12.1541, -25.3546) projected
  line L1317 (12.1541, -25.3546) -> (12.1541, -26.0046) projected
  line L1318 (12.1541, -26.0046) -> (11.8439, -26.0046) projected
  arc A70 (12.1166, -26.7296) -> (11.8439, -26.0046) centre (11.0166, -26.7296) ccw projected
  line L1319 (12.1166, -26.7296) -> (12.1166, -32.6296) projected
  arc A71 (11.9218, -33.2546) -> (12.1166, -32.6296) centre (11.0166, -32.6296) ccw projected
  line L1320 (11.9218, -33.2546) -> (12.1541, -33.2546) projected
  line L1321 (12.1541, -33.2546) -> (12.1541, -33.9046) projected
  line L1322 (12.1541, -33.9046) -> (10.5541, -33.9046) projected
  line L1323 (10.5541, -33.9046) -> (10.5541, -33.6276) projected
  arc A72 (9.9166, -32.6296) -> (10.5541, -33.6276) centre (11.0166, -32.6296) ccw projected
  line L1324 (9.9166, -32.6296) -> (9.6891, -32.6296) projected
  line L1325 (9.6891, -32.6296) -> (9.6891, -32.2296) projected
  line L1326 (9.6891, -32.2296) -> (9.9166, -32.2296) projected
  line L1327 (9.9166, -32.2296) -> (9.9166, -31.8296) projected
  line L1328 (9.9166, -31.8296) -> (9.6891, -31.8296) projected
  line L1329 (9.6891, -31.8296) -> (9.6891, -31.4296) projected
  line L1330 (9.6891, -31.4296) -> (9.9166, -31.4296) projected
  arc A73 (10.5583, 3.7704) -> (11.4749, 3.7704) centre (11.0166, 4.7704) ccw projected
  line L1331 (10.5583, 3.7704) -> (10.3966, 3.7704) projected
  line L1332 (10.3966, 3.7704) -> (10.3966, 3.8618) projected
  arc A74 (9.9166, 4.7704) -> (10.3966, 3.8618) centre (11.0166, 4.7704) ccw projected
  line L1333 (9.9166, 4.7704) -> (9.9166, 5.0454) projected
  line L1334 (9.9166, 5.0454) -> (9.5316, 5.0454) projected
  line L1335 (9.5316, 5.0454) -> (9.5316, 5.4454) projected
  line L1336 (9.5316, 5.4454) -> (9.9166, 5.4454) projected
  line L1337 (9.9166, 5.4454) -> (9.9166, 5.8454) projected
  line L1338 (9.9166, 5.8454) -> (9.5316, 5.8454) projected
  line L1339 (9.5316, 5.8454) -> (9.5316, 6.2454) projected
  line L1340 (9.5316, 6.2454) -> (9.9166, 6.2454) projected
  line L1341 (9.9166, 6.2454) -> (9.9166, 6.6454) projected
  line L1342 (9.9166, 6.6454) -> (9.5316, 6.6454) projected
  line L1343 (9.5316, 6.6454) -> (9.5316, 7.0454) projected
  line L1344 (9.5316, 7.0454) -> (9.9166, 7.0454) projected
  line L1345 (9.9166, 7.0454) -> (9.9166, 7.4454) projected
  line L1346 (9.9166, 7.4454) -> (9.5316, 7.4454) projected
  line L1347 (9.5316, 7.4454) -> (9.5316, 7.8454) projected
  line L1348 (9.5316, 7.8454) -> (9.9166, 7.8454) projected
  line L1349 (9.9166, 7.8454) -> (9.9166, 8.2454) projected
  line L1350 (9.9166, 8.2454) -> (9.5316, 8.2454) projected
  line L1351 (9.5316, 8.2454) -> (9.5316, 8.6454) projected
  line L1352 (9.5316, 8.6454) -> (9.9166, 8.6454) projected
  line L1353 (9.9166, 8.6454) -> (9.9166, 9.0454) projected
  line L1354 (9.9166, 9.0454) -> (9.5316, 9.0454) projected
  line L1355 (9.5316, 9.0454) -> (9.5316, 9.4454) projected
  line L1356 (9.5316, 9.4454) -> (9.9166, 9.4454) projected
  line L1357 (9.9166, 9.4454) -> (9.9166, 9.8454) projected
  line L1358 (9.9166, 9.8454) -> (9.5316, 9.8454) projected
  line L1359 (9.5316, 9.8454) -> (9.5316, 10.2454) projected
  line L1360 (9.5316, 10.2454) -> (9.9166, 10.2454) projected
  line L1361 (9.9166, 10.2454) -> (9.9166, 10.6454) projected
  line L1362 (9.9166, 10.6454) -> (9.5316, 10.6454) projected
  line L1363 (9.5316, 10.6454) -> (9.5316, 11.0454) projected
  line L1364 (9.5316, 11.0454) -> (9.9825, 11.0454) projected
  arc A75 (10.5583, 11.6704) -> (9.9825, 11.0454) centre (11.0166, 10.6704) ccw projected
  line L1365 (10.5583, 11.6704) -> (10.3966, 11.6704) projected
  line L1366 (10.3966, 11.6704) -> (10.3966, 12.3204) projected
  line L1367 (10.3966, 12.3204) -> (11.9966, 12.3204) projected
  line L1368 (11.9966, 12.3204) -> (11.9966, 11.6704) projected
  line L1369 (11.9966, 11.6704) -> (11.4749, 11.6704) projected
  arc A76 (12.0716, 10.9818) -> (11.4749, 11.6704) centre (11.0166, 10.6704) ccw projected
  line L1370 (12.0716, 10.9818) -> (12.0716, 11.0454) projected
  line L1371 (12.0716, 11.0454) -> (12.8616, 11.0454) projected
  line L1372 (12.8616, 11.0454) -> (12.8616, 10.6454) projected
  line L1373 (12.8616, 10.6454) -> (12.1166, 10.6454) projected
  line L1374 (12.1166, 10.6454) -> (12.1166, 10.2454) projected
  line L1375 (12.1166, 10.2454) -> (12.8616, 10.2454) projected
  line L1376 (12.8616, 10.2454) -> (12.8616, 9.8454) projected
  line L1377 (12.8616, 9.8454) -> (12.1166, 9.8454) projected
  line L1378 (12.1166, 9.8454) -> (12.1166, 9.4454) projected
  line L1379 (12.1166, 9.4454) -> (12.8616, 9.4454) projected
  line L1380 (12.8616, 9.4454) -> (12.8616, 9.0454) projected
  line L1381 (12.8616, 9.0454) -> (12.1166, 9.0454) projected
  line L1382 (12.1166, 9.0454) -> (12.1166, 8.6454) projected
  line L1383 (12.1166, 8.6454) -> (12.8616, 8.6454) projected
  line L1384 (12.8616, 8.6454) -> (12.8616, 8.2454) projected
  line L1385 (12.8616, 8.2454) -> (12.1166, 8.2454) projected
  line L1386 (12.1166, 8.2454) -> (12.1166, 7.8454) projected
  line L1387 (12.1166, 7.8454) -> (12.8616, 7.8454) projected
  line L1388 (12.8616, 7.8454) -> (12.8616, 7.4454) projected
  line L1389 (12.8616, 7.4454) -> (12.1166, 7.4454) projected
  line L1390 (12.1166, 7.4454) -> (12.1166, 7.0454) projected
  line L1391 (12.1166, 7.0454) -> (12.8616, 7.0454) projected
  line L1392 (12.8616, 7.0454) -> (12.8616, 6.6454) projected
  line L1393 (12.8616, 6.6454) -> (12.1166, 6.6454) projected
  line L1394 (12.1166, 6.6454) -> (12.1166, 6.2454) projected
  line L1395 (12.1166, 6.2454) -> (12.8616, 6.2454) projected
  line L1396 (12.8616, 6.2454) -> (12.8616, 5.8454) projected
  line L1397 (12.8616, 5.8454) -> (12.1166, 5.8454) projected
  line L1398 (12.1166, 5.8454) -> (12.1166, 5.4454) projected
  line L1399 (12.1166, 5.4454) -> (12.8616, 5.4454) projected
  line L1400 (12.8616, 5.4454) -> (12.8616, 5.0454) projected
  line L1401 (12.8616, 5.0454) -> (12.1166, 5.0454) projected
  line L1402 (12.1166, 5.0454) -> (12.1166, 4.7704) projected
  arc A77 (11.9966, 4.2708) -> (12.1166, 4.7704) centre (11.0166, 4.7704) ccw projected
  line L1403 (11.9966, 4.2708) -> (11.9966, 3.7704) projected
  line L1404 (11.9966, 3.7704) -> (11.4749, 3.7704) projected
  line L1405 (9.9166, 24.7954) -> (9.9166, 25.1954) projected
  line L1406 (9.9166, 25.1954) -> (9.7466, 25.1954) projected
  line L1407 (9.7466, 25.1954) -> (9.7466, 25.5954) projected
  line L1408 (9.7466, 25.5954) -> (9.9166, 25.5954) projected
  line L1409 (9.9166, 25.5954) -> (9.9166, 25.9954) projected
  line L1410 (9.9166, 25.9954) -> (9.7466, 25.9954) projected
  line L1411 (9.7466, 25.9954) -> (9.7466, 26.3954) projected
  line L1412 (9.7466, 26.3954) -> (9.9166, 26.3954) projected
  line L1413 (9.9166, 26.3954) -> (9.9166, 26.7954) projected
  line L1414 (9.9166, 26.7954) -> (9.7466, 26.7954) projected
  line L1415 (9.7466, 26.7954) -> (9.7466, 27.1954) projected
  line L1416 (9.7466, 27.1954) -> (9.9166, 27.1954) projected
  line L1417 (9.9166, 27.1954) -> (9.9166, 27.5954) projected
  line L1418 (9.9166, 27.5954) -> (9.7466, 27.5954) projected
  line L1419 (9.7466, 27.5954) -> (9.7466, 27.9954) projected
  line L1420 (9.7466, 27.9954) -> (9.9166, 27.9954) projected
  line L1421 (9.9166, 27.9954) -> (9.9166, 28.3954) projected
  line L1422 (9.9166, 28.3954) -> (9.7466, 28.3954) projected
  line L1423 (9.7466, 28.3954) -> (9.7466, 28.7954) projected
  line L1424 (9.7466, 28.7954) -> (9.9166, 28.7954) projected
  line L1425 (9.9166, 28.7954) -> (9.9166, 29.1954) projected
  line L1426 (9.9166, 29.1954) -> (9.7466, 29.1954) projected
  line L1427 (9.7466, 29.1954) -> (9.7466, 29.5954) projected
  line L1428 (9.7466, 29.5954) -> (9.9399, 29.5954) projected
  arc A78 (10.6116, 30.3931) -> (9.9399, 29.5954) centre (11.0166, 29.3704) ccw projected
  line L1429 (10.6116, 30.3931) -> (10.6116, 30.8704) projected
  line L1430 (10.6116, 30.8704) -> (12.2116, 30.8704) projected
  line L1431 (12.2116, 30.8704) -> (12.2116, 30.2204) projected
  line L1432 (12.2116, 30.2204) -> (11.7148, 30.2204) projected
  arc A79 (12.1166, 29.3704) -> (11.7148, 30.2204) centre (11.0166, 29.3704) ccw projected
  line L1433 (12.1166, 29.3704) -> (12.1166, 23.4704) projected
  arc A80 (11.9964, 22.9704) -> (12.1166, 23.4704) centre (11.0166, 23.4704) ccw projected
  line L1434 (11.9964, 22.9704) -> (12.2116, 22.9704) projected
  line L1435 (12.2116, 22.9704) -> (12.2116, 22.3204) projected
  line L1436 (12.2116, 22.3204) -> (10.6116, 22.3204) projected
  line L1437 (10.6116, 22.3204) -> (10.6116, 22.4477) projected
  arc A81 (9.9166, 23.4704) -> (10.6116, 22.4477) centre (11.0166, 23.4704) ccw projected
  line L1438 (9.9166, 23.4704) -> (9.9166, 23.5954) projected
  line L1439 (9.9166, 23.5954) -> (9.7466, 23.5954) projected
  line L1440 (9.7466, 23.5954) -> (9.7466, 23.9954) projected
  line L1441 (9.7466, 23.9954) -> (9.9166, 23.9954) projected
  line L1442 (9.9166, 23.9954) -> (9.9166, 24.3954) projected
  line L1443 (9.9166, 24.3954) -> (9.7466, 24.3954) projected
  line L1444 (9.7466, 24.3954) -> (9.7466, 24.7954) projected
  line L1445 (9.7466, 24.7954) -> (9.9166, 24.7954) projected
  line L1446 (28.6166, -31.5296) -> (28.6166, -31.1296) projected
  line L1447 (28.6166, -31.1296) -> (28.5141, -31.1296) projected
  line L1448 (28.5141, -31.1296) -> (28.5141, -30.7296) projected
  line L1449 (28.5141, -30.7296) -> (28.6166, -30.7296) projected
  line L1450 (28.6166, -30.7296) -> (28.6166, -30.3296) projected
  line L1451 (28.6166, -30.3296) -> (28.5141, -30.3296) projected
  line L1452 (28.5141, -30.3296) -> (28.5141, -29.9296) projected
  line L1453 (28.5141, -29.9296) -> (28.6166, -29.9296) projected
  line L1454 (28.6166, -29.9296) -> (28.6166, -29.5296) projected
  line L1455 (28.6166, -29.5296) -> (28.5141, -29.5296) projected
  line L1456 (28.5141, -29.5296) -> (28.5141, -29.1296) projected
  line L1457 (28.5141, -29.1296) -> (28.6166, -29.1296) projected
  line L1458 (28.6166, -29.1296) -> (28.6166, -28.7296) projected
  line L1459 (28.6166, -28.7296) -> (28.5141, -28.7296) projected
  line L1460 (28.5141, -28.7296) -> (28.5141, -28.3296) projected
  line L1461 (28.5141, -28.3296) -> (28.6166, -28.3296) projected
  line L1462 (28.6166, -28.3296) -> (28.6166, -27.9296) projected
  line L1463 (28.6166, -27.9296) -> (28.5141, -27.9296) projected
  line L1464 (28.5141, -27.9296) -> (28.5141, -27.5296) projected
  line L1465 (28.5141, -27.5296) -> (28.6166, -27.5296) projected
  line L1466 (28.6166, -27.5296) -> (28.6166, -27.1296) projected
  line L1467 (28.6166, -27.1296) -> (28.5141, -27.1296) projected
  line L1468 (28.5141, -27.1296) -> (28.5141, -26.7296) projected
  line L1469 (28.5141, -26.7296) -> (28.6166, -26.7296) projected
  arc A82 (29.3791, -25.6827) -> (28.6166, -26.7296) centre (29.7166, -26.7296) ccw projected
  line L1470 (29.3791, -25.6827) -> (29.3791, -25.4546) projected
  line L1471 (29.3791, -25.4546) -> (30.9791, -25.4546) projected
  line L1472 (30.9791, -25.4546) -> (30.9791, -26.1046) projected
  line L1473 (30.9791, -26.1046) -> (30.6218, -26.1046) projected
  arc A83 (30.8166, -26.7296) -> (30.6218, -26.1046) centre (29.7166, -26.7296) ccw projected
  line L1474 (30.8166, -26.7296) -> (30.8166, -32.6296) projected
  arc A84 (30.5439, -33.3546) -> (30.8166, -32.6296) centre (29.7166, -32.6296) ccw projected
  line L1475 (30.5439, -33.3546) -> (30.9791, -33.3546) projected
  line L1476 (30.9791, -33.3546) -> (30.9791, -34.0046) projected
  line L1477 (30.9791, -34.0046) -> (29.3791, -34.0046) projected
  line L1478 (29.3791, -34.0046) -> (29.3791, -33.6765) projected
  arc A85 (28.6212, -32.7296) -> (29.3791, -33.6765) centre (29.7166, -32.6296) ccw projected
  line L1479 (28.6212, -32.7296) -> (28.5141, -32.7296) projected
  line L1480 (28.5141, -32.7296) -> (28.5141, -32.3296) projected
  line L1481 (28.5141, -32.3296) -> (28.6166, -32.3296) projected
  line L1482 (28.6166, -32.3296) -> (28.6166, -31.9296) projected
  line L1483 (28.6166, -31.9296) -> (28.5141, -31.9296) projected
  line L1484 (28.5141, -31.9296) -> (28.5141, -31.5296) projected
  line L1485 (28.5141, -31.5296) -> (28.6166, -31.5296) projected
  arc A86 (30.4716, -14.7296) -> (30.8166, -13.9296) centre (29.7166, -13.9296) ccw projected
  line L1486 (30.4716, -14.7296) -> (31.0941, -14.7296) projected
  line L1487 (31.0941, -14.7296) -> (31.0941, -15.3796) projected
  line L1488 (31.0941, -15.3796) -> (29.4941, -15.3796) projected
  line L1489 (29.4941, -15.3796) -> (29.4941, -15.0069) projected
  arc A87 (28.6306, -14.1046) -> (29.4941, -15.0069) centre (29.7166, -13.9296) ccw projected
  line L1490 (28.6306, -14.1046) -> (28.6291, -14.1046) projected
  line L1491 (28.6291, -14.1046) -> (28.6291, -14.095) projected
  arc A88 (28.6166, -13.9296) -> (28.6291, -14.095) centre (29.7166, -13.9296) ccw projected
  line L1492 (28.6166, -13.9296) -> (28.6166, -8.0296) projected
  arc A89 (29.4941, -6.9523) -> (28.6166, -8.0296) centre (29.7166, -8.0296) ccw projected
  line L1493 (29.4941, -6.9523) -> (29.4941, -6.8296) projected
  line L1494 (29.4941, -6.8296) -> (31.0941, -6.8296) projected
  line L1495 (31.0941, -6.8296) -> (31.0941, -7.4796) projected
  line L1496 (31.0941, -7.4796) -> (30.6692, -7.4796) projected
  arc A90 (30.8166, -8.0296) -> (30.6692, -7.4796) centre (29.7166, -8.0296) ccw projected
  line L1497 (30.8166, -8.0296) -> (30.8166, -13.9296) projected
  line L1498 (28.6166, 6.1454) -> (28.6166, 6.5454) projected
  line L1499 (28.6166, 6.5454) -> (28.3566, 6.5454) projected
  line L1500 (28.3566, 6.5454) -> (28.3566, 6.9454) projected
  line L1501 (28.3566, 6.9454) -> (28.6166, 6.9454) projected
  line L1502 (28.6166, 6.9454) -> (28.6166, 7.3454) projected
  line L1503 (28.6166, 7.3454) -> (28.3566, 7.3454) projected
  line L1504 (28.3566, 7.3454) -> (28.3566, 7.7454) projected
  line L1505 (28.3566, 7.7454) -> (28.6166, 7.7454) projected
  line L1506 (28.6166, 7.7454) -> (28.6166, 8.1454) projected
  line L1507 (28.6166, 8.1454) -> (28.3566, 8.1454) projected
  line L1508 (28.3566, 8.1454) -> (28.3566, 8.5454) projected
  line L1509 (28.3566, 8.5454) -> (28.6166, 8.5454) projected
  line L1510 (28.6166, 8.5454) -> (28.6166, 8.9454) projected
  line L1511 (28.6166, 8.9454) -> (28.3566, 8.9454) projected
  line L1512 (28.3566, 8.9454) -> (28.3566, 9.3454) projected
  line L1513 (28.3566, 9.3454) -> (28.6166, 9.3454) projected
  line L1514 (28.6166, 9.3454) -> (28.6166, 9.7454) projected
  line L1515 (28.6166, 9.7454) -> (28.3566, 9.7454) projected
  line L1516 (28.3566, 9.7454) -> (28.3566, 10.1454) projected
  line L1517 (28.3566, 10.1454) -> (28.6166, 10.1454) projected
  line L1518 (28.6166, 10.1454) -> (28.6166, 10.5454) projected
  line L1519 (28.6166, 10.5454) -> (28.3566, 10.5454) projected
  line L1520 (28.3566, 10.5454) -> (28.3566, 10.9454) projected
  line L1521 (28.3566, 10.9454) -> (28.6515, 10.9454) projected
  arc A91 (29.2216, 11.6527) -> (28.6515, 10.9454) centre (29.7166, 10.6704) ccw projected
  line L1522 (29.2216, 11.6527) -> (29.2216, 12.2204) projected
  line L1523 (29.2216, 12.2204) -> (30.8216, 12.2204) projected
  line L1524 (30.8216, 12.2204) -> (30.8216, 11.5704) projected
  line L1525 (30.8216, 11.5704) -> (30.3491, 11.5704) projected
  arc A92 (30.8166, 10.6704) -> (30.3491, 11.5704) centre (29.7166, 10.6704) ccw projected
  line L1526 (30.8166, 10.6704) -> (30.8166, 4.7704) projected
  arc A93 (30.7203, 4.3204) -> (30.8166, 4.7704) centre (29.7166, 4.7704) ccw projected
  line L1527 (30.7203, 4.3204) -> (30.8216, 4.3204) projected
  line L1528 (30.8216, 4.3204) -> (30.8216, 3.6704) projected
  line L1529 (30.8216, 3.6704) -> (29.7166, 3.6704) projected
  line L1530 (29.7166, 3.6704) -> (29.2216, 3.6704) projected
  line L1531 (29.2216, 3.6704) -> (29.2216, 3.7881) projected
  arc A94 (28.6166, 4.7704) -> (29.2216, 3.7881) centre (29.7166, 4.7704) ccw projected
  line L1532 (28.6166, 4.7704) -> (28.6166, 4.9454) projected
  line L1533 (28.6166, 4.9454) -> (28.3566, 4.9454) projected
  line L1534 (28.3566, 4.9454) -> (28.3566, 5.3454) projected
  line L1535 (28.3566, 5.3454) -> (28.6166, 5.3454) projected
  line L1536 (28.6166, 5.3454) -> (28.6166, 5.7454) projected
  line L1537 (28.6166, 5.7454) -> (28.3566, 5.7454) projected
  line L1538 (28.3566, 5.7454) -> (28.3566, 6.1454) projected
  line L1539 (28.3566, 6.1454) -> (28.6166, 6.1454) projected
  arc A95 (29.4834, 22.3954) -> (29.9498, 22.3954) centre (29.7166, 23.4704) ccw projected
  line L1540 (29.4834, 22.3954) -> (29.4191, 22.3954) projected
  line L1541 (29.4191, 22.3954) -> (29.4191, 22.4114) projected
  arc A96 (28.6166, 23.4704) -> (29.4191, 22.4114) centre (29.7166, 23.4704) ccw projected
  line L1542 (28.6166, 23.4704) -> (28.6166, 23.6704) projected
  line L1543 (28.6166, 23.6704) -> (28.5541, 23.6704) projected
  line L1544 (28.5541, 23.6704) -> (28.5541, 24.0704) projected
  line L1545 (28.5541, 24.0704) -> (28.6166, 24.0704) projected
  line L1546 (28.6166, 24.0704) -> (28.6166, 24.4704) projected
  line L1547 (28.6166, 24.4704) -> (28.5541, 24.4704) projected
  line L1548 (28.5541, 24.4704) -> (28.5541, 24.8704) projected
  line L1549 (28.5541, 24.8704) -> (28.6166, 24.8704) projected
  line L1550 (28.6166, 24.8704) -> (28.6166, 25.2704) projected
  line L1551 (28.6166, 25.2704) -> (28.5541, 25.2704) projected
  line L1552 (28.5541, 25.2704) -> (28.5541, 25.6704) projected
  line L1553 (28.5541, 25.6704) -> (28.6166, 25.6704) projected
  line L1554 (28.6166, 25.6704) -> (28.6166, 26.0704) projected
  line L1555 (28.6166, 26.0704) -> (28.5541, 26.0704) projected
  line L1556 (28.5541, 26.0704) -> (28.5541, 26.4704) projected
  line L1557 (28.5541, 26.4704) -> (28.6166, 26.4704) projected
  line L1558 (28.6166, 26.4704) -> (28.6166, 26.8704) projected
  line L1559 (28.6166, 26.8704) -> (28.5541, 26.8704) projected
  line L1560 (28.5541, 26.8704) -> (28.5541, 27.2704) projected
  line L1561 (28.5541, 27.2704) -> (28.6166, 27.2704) projected
  line L1562 (28.6166, 27.2704) -> (28.6166, 27.6704) projected
  line L1563 (28.6166, 27.6704) -> (28.5541, 27.6704) projected
  line L1564 (28.5541, 27.6704) -> (28.5541, 28.0704) projected
  line L1565 (28.5541, 28.0704) -> (28.6166, 28.0704) projected
  line L1566 (28.6166, 28.0704) -> (28.6166, 28.4704) projected
  line L1567 (28.6166, 28.4704) -> (28.5541, 28.4704) projected
  line L1568 (28.5541, 28.4704) -> (28.5541, 28.8704) projected
  line L1569 (28.5541, 28.8704) -> (28.6166, 28.8704) projected
  line L1570 (28.6166, 28.8704) -> (28.6166, 29.2704) projected
  line L1571 (28.6166, 29.2704) -> (28.5541, 29.2704) projected
  line L1572 (28.5541, 29.2704) -> (28.5541, 29.6704) projected
  line L1573 (28.5541, 29.6704) -> (28.6583, 29.6704) projected
  arc A97 (29.4191, 30.4294) -> (28.6583, 29.6704) centre (29.7166, 29.3704) ccw projected
  line L1574 (29.4191, 30.4294) -> (29.4191, 30.9454) projected
  line L1575 (29.4191, 30.9454) -> (31.0191, 30.9454) projected
  line L1576 (31.0191, 30.9454) -> (31.0191, 30.2954) projected
  line L1577 (31.0191, 30.2954) -> (30.3119, 30.2954) projected
  arc A98 (30.8166, 29.3704) -> (30.3119, 30.2954) centre (29.7166, 29.3704) ccw projected
  line L1578 (30.8166, 29.3704) -> (30.8166, 23.4704) projected
  arc A99 (30.7312, 23.0454) -> (30.8166, 23.4704) centre (29.7166, 23.4704) ccw projected
  line L1579 (30.7312, 23.0454) -> (31.0191, 23.0454) projected
  line L1580 (31.0191, 23.0454) -> (31.0191, 22.3954) projected
  line L1581 (31.0191, 22.3954) -> (29.9498, 22.3954) projected
  line L1582 (47.3166, 24.8454) -> (47.3166, 25.2454) projected
  line L1583 (47.3166, 25.2454) -> (47.3091, 25.2454) projected
  line L1584 (47.3091, 25.2454) -> (47.3091, 25.6454) projected
  line L1585 (47.3091, 25.6454) -> (47.3166, 25.6454) projected
  line L1586 (47.3166, 25.6454) -> (47.3166, 26.0454) projected
  line L1587 (47.3166, 26.0454) -> (47.3091, 26.0454) projected
  line L1588 (47.3091, 26.0454) -> (47.3091, 26.4454) projected
  line L1589 (47.3091, 26.4454) -> (47.3166, 26.4454) projected
  line L1590 (47.3166, 26.4454) -> (47.3166, 26.8454) projected
  line L1591 (47.3166, 26.8454) -> (47.3091, 26.8454) projected
  line L1592 (47.3091, 26.8454) -> (47.3091, 27.2454) projected
  line L1593 (47.3091, 27.2454) -> (47.3166, 27.2454) projected
  line L1594 (47.3166, 27.2454) -> (47.3166, 27.6454) projected
  line L1595 (47.3166, 27.6454) -> (47.3091, 27.6454) projected
  line L1596 (47.3091, 27.6454) -> (47.3091, 28.0454) projected
  line L1597 (47.3091, 28.0454) -> (47.3166, 28.0454) projected
  line L1598 (47.3166, 28.0454) -> (47.3166, 28.4454) projected
  line L1599 (47.3166, 28.4454) -> (47.3091, 28.4454) projected
  line L1600 (47.3091, 28.4454) -> (47.3091, 28.8454) projected
  line L1601 (47.3091, 28.8454) -> (47.3166, 28.8454) projected
  line L1602 (47.3166, 28.8454) -> (47.3166, 29.2454) projected
  line L1603 (47.3166, 29.2454) -> (47.3091, 29.2454) projected
  line L1604 (47.3091, 29.2454) -> (47.3091, 29.6454) projected
  line L1605 (47.3091, 29.6454) -> (47.3515, 29.6454) projected
  arc A100 (48.1741, 30.4433) -> (47.3515, 29.6454) centre (48.4166, 29.3704) ccw projected
  line L1606 (48.1741, 30.4433) -> (48.1741, 30.9204) projected
  line L1607 (48.1741, 30.9204) -> (49.7741, 30.9204) projected
  line L1608 (49.7741, 30.9204) -> (49.7741, 30.2704) projected
  line L1609 (49.7741, 30.2704) -> (49.0491, 30.2704) projected
  arc A101 (49.5166, 29.3704) -> (49.0491, 30.2704) centre (48.4166, 29.3704) ccw projected
  line L1610 (49.5166, 29.3704) -> (49.5166, 23.4704) projected
  arc A102 (49.4203, 23.0204) -> (49.5166, 23.4704) centre (48.4166, 23.4704) ccw projected
  line L1611 (49.4203, 23.0204) -> (49.7741, 23.0204) projected
  line L1612 (49.7741, 23.0204) -> (49.7741, 22.3704) projected
  line L1613 (49.7741, 22.3704) -> (48.4166, 22.3704) projected
  line L1614 (48.4166, 22.3704) -> (48.1741, 22.3704) projected
  line L1615 (48.1741, 22.3704) -> (48.1741, 22.3975) projected
  arc A103 (47.3166, 23.4704) -> (48.1741, 22.3975) centre (48.4166, 23.4704) ccw projected
  line L1616 (47.3166, 23.4704) -> (47.3166, 23.6454) projected
  line L1617 (47.3166, 23.6454) -> (47.3091, 23.6454) projected
  line L1618 (47.3091, 23.6454) -> (47.3091, 24.0454) projected
  line L1619 (47.3091, 24.0454) -> (47.3166, 24.0454) projected
  line L1620 (47.3166, 24.0454) -> (47.3166, 24.4454) projected
  line L1621 (47.3166, 24.4454) -> (47.3091, 24.4454) projected
  line L1622 (47.3091, 24.4454) -> (47.3091, 24.8454) projected
  line L1623 (47.3091, 24.8454) -> (47.3166, 24.8454) projected
  line L1624 (72.421, 51.4152) -> (-72.421, 51.4152)
  line L1625 (-72.421, 51.4152) -> (-72.421, -51.4152)
  line L1626 (-72.421, -51.4152) -> (72.421, -51.4152)
  line L1627 (72.421, -51.4152) -> (72.421, 51.4152)
  line L1628 (68.921, 47.9152) -> (-68.921, 47.9152)
  line L1629 (-68.921, 47.9152) -> (-68.921, -47.9152)
  line L1630 (-68.921, -47.9152) -> (68.921, -47.9152)
  line L1631 (68.921, -47.9152) -> (68.921, 47.9152)
  circle A104 centre (68.921, 47.9152) radius 1.4
  circle A105 centre (68.921, -47.9152) radius 1.4
  circle A106 centre (-68.921, -47.9152) radius 1.4
  circle A107 centre (-68.921, 47.9152) radius 1.5
  point P0 (0, 0)
  dimension "d0" = 6
  dimension "d1" = 3.5
  dimension "d2" = 2.8
  dimension "d3" = 2.8
  dimension "d4" = 2.8
  dimension "d5" = 3
  constraints: 16 end point, 4 centre point, 4 coincident, 6 other
  measures "d0" distance between parallel lines of L675 L1627
  measures "d1" distance between parallel lines of L1627 L1631
  measures "d2" diameter of A104
  measures "d3" diameter of A105
  measures "d4" diameter of A106
  measures "d5" diameter of A107